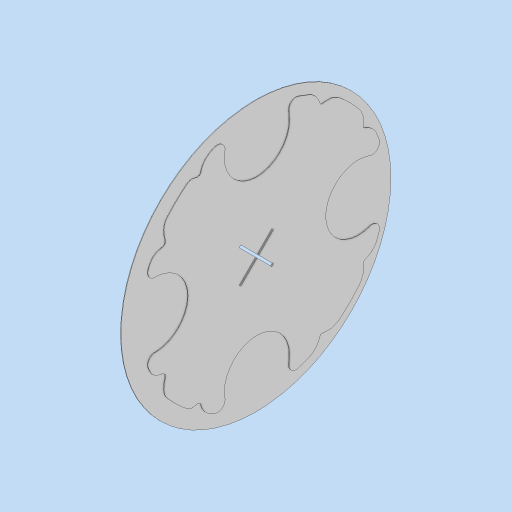
# Autodesk Inventor part: Sticker1
Saved by Autodesk Inventor 2024 (Build 280153000, 153)
## iProperties
Created: 2025-01-25
Part Number: Sticker1
Material: Generic
Document SubType Name: Modeling
Designer: Dmitry
Density: 1 g/cm^3
Appearance: Default
Author: Dmitry
Autodesk Inventor part; units mm, degrees
(part 1 of 2)
ref_plane "YZ Plane" through (0, 0, 0) normal (1, 0, 0) x (0, 1, 0)
ref_plane "XZ Plane" through (0, 0, 0) normal (0, 1, 0) x (-1, 0, 0)
ref_plane "XY Plane" through (0, 0, 0) normal (0, 0, 1) x (1, 0, 0)
sketch "Sketch1" plane through (0, 0, 0) normal (1, 0, 0) x (0, 1, 0)
  line L0 (61.7061, -10.6192) -> (60.2494, -12.386)
  line L1 (60.2494, -12.386) -> (59.1486, -14.4129)
  line L2 (59.1486, -14.4129) -> (58.4523, -16.6524)
  line L3 (58.4523, -16.6524) -> (58.211, -18.4561)
  line L4 (58.211, -18.4561) -> (58.211, -19.0583)
  line L5 (58.211, -19.0583) -> (58.211, -19.6593)
  line L6 (58.211, -19.6593) -> (58.4523, -21.4632)
  line L7 (58.4523, -21.4632) -> (59.1486, -23.7037)
  line L8 (59.1486, -23.7037) -> (60.2494, -25.7309)
  line L9 (60.2494, -25.7309) -> (61.7061, -27.4975)
  line L10 (61.7061, -39.6202) -> (60.2494, -41.3868)
  line L11 (60.2494, -41.3868) -> (59.1486, -43.4139)
  line L12 (59.1486, -43.4139) -> (58.4523, -45.6533)
  line L13 (58.4523, -45.6533) -> (58.211, -47.4571)
  line L14 (58.211, -47.4571) -> (58.211, -48.0593)
  line L15 (58.211, -48.0593) -> (58.211, -48.6601)
  line L16 (58.211, -48.6601) -> (58.4523, -50.464)
  line L17 (58.4523, -50.464) -> (59.1486, -52.7033)
  line L18 (59.1486, -52.7033) -> (60.2494, -54.7304)
  line L19 (60.2494, -54.7304) -> (61.7061, -56.497)
  line L20 (61.7061, 18.3803) -> (60.2494, 16.6135)
  line L21 (60.2494, 16.6135) -> (59.1486, 14.5863)
  line L22 (59.1486, 14.5863) -> (58.4523, 12.347)
  line L23 (58.4523, 12.347) -> (58.211, 10.5431)
  line L24 (58.211, 10.5431) -> (58.211, 9.9411)
  line L25 (58.211, 9.9411) -> (58.211, 9.3402)
  line L26 (58.211, 9.3402) -> (58.4523, 7.5363)
  line L27 (58.4523, 7.5363) -> (59.1486, 5.297)
  line L28 (59.1486, 5.297) -> (60.2494, 3.2701)
  line L29 (60.2494, 3.2701) -> (61.7061, 1.5032)
  line L30 (-65.1162, -39.6422) -> (-65.1135, -39.6381)
  line L31 (-65.1135, -39.6381) -> (-65.0777, -39.6023)
  line L32 (-65.0777, -39.6023) -> (-65.0735, -39.5995)
  line L33 (-65.0735, -39.5995) -> (-64.7194, -39.2412)
  line L34 (-64.7194, -39.2412) -> (-63.3482, -38.4723)
  line L35 (-63.3482, -38.4723) -> (-61.3997, -38.1637)
  line L36 (-61.3997, -38.1637) -> (-59.5007, -38.6666)
  line L37 (-59.5007, -38.6666) -> (-58.2302, -39.5816)
  line L38 (-58.2302, -39.5816) -> (-57.9229, -39.9771)
  line L39 (-57.9229, -39.9771) -> (-57.4888, -40.5366)
  line L40 (-57.4888, -40.5366) -> (-55.2495, -43.4098)
  line L41 (-55.2495, -43.4098) -> (-53.1783, -46.0363)
  line L42 (-53.1783, -46.0363) -> (-52.8283, -46.4746)
  line L43 (-52.8283, -46.4746) -> (-52.4672, -46.9265)
  line L44 (-52.4672, -46.9265) -> (-51.3813, -48.2853)
  line L45 (-51.3813, -48.2853) -> (-50.1039, -49.8893)
  line L46 (-50.1039, -49.8893) -> (-49.1268, -51.1364)
  line L47 (-49.1268, -51.1364) -> (-48.6749, -51.7276)
  line L48 (-48.6749, -51.7276) -> (-48.5784, -51.871)
  line L49 (-48.5784, -51.871) -> (-48.4159, -52.1093)
  line L50 (-48.4159, -52.1093) -> (-48.2889, -52.2968)
  line L51 (-48.2889, -52.2968) -> (-47.9058, -52.8618)
  line L52 (-47.9058, -52.8618) -> (-47.2886, -53.8057)
  line L53 (-47.2886, -53.8057) -> (-46.6341, -54.8682)
  line L54 (-46.6341, -54.8682) -> (-46.0138, -55.9775)
  line L55 (-46.0138, -55.9775) -> (-45.4999, -57.0593)
  line L56 (-45.4999, -57.0593) -> (-45.1621, -58.0432)
  line L57 (-45.1621, -58.0432) -> (-45.074, -58.8576)
  line L58 (-45.074, -58.8576) -> (-45.2051, -59.3261)
  line L59 (-45.2051, -59.3261) -> (-45.3028, -59.4281)
  line L60 (-45.3028, -59.4281) -> (-45.3153, -59.4405)
  line L61 (-45.3153, -59.4405) -> (-45.5137, -59.6321)
  line L62 (-45.5137, -59.6321) -> (-46.7098, -59.5907)
  line L63 (-46.7098, -59.5907) -> (-48.7809, -58.7446)
  line L64 (-48.7809, -58.7446) -> (-50.9527, -57.4727)
  line L65 (-50.9527, -57.4727) -> (-52.2302, -56.6321)
  line L66 (-52.2302, -56.6321) -> (-52.6505, -56.3468)
  line L67 (-52.6505, -56.3468) -> (-52.8903, -56.1828)
  line L68 (-52.8903, -56.1828) -> (-53.0322, -56.0864)
  line L69 (-53.0322, -56.0864) -> (-53.622, -55.6357)
  line L70 (-53.622, -55.6357) -> (-54.8636, -54.6615)
  line L71 (-54.8636, -54.6615) -> (-56.4635, -53.3895)
  line L72 (-56.4635, -53.3895) -> (-57.8168, -52.3064)
  line L73 (-57.8168, -52.3064) -> (-58.2674, -51.9467)
  line L74 (-58.2674, -51.9467) -> (-58.7056, -51.5967)
  line L75 (-58.7056, -51.5967) -> (-61.339, -49.52)
  line L76 (-61.339, -49.52) -> (-64.2219, -47.2738)
  line L77 (-64.2219, -47.2738) -> (-64.7841, -46.8383)
  line L78 (-64.7841, -46.8383) -> (-65.1796, -46.531)
  line L79 (-65.1796, -46.531) -> (-66.0946, -45.2591)
  line L80 (-66.0946, -45.2591) -> (-66.5976, -43.3616)
  line L81 (-66.5976, -43.3616) -> (-66.289, -41.413)
  line L82 (-66.289, -41.413) -> (-65.52, -40.0419)
  line L83 (-65.52, -40.0419) -> (-65.1617, -39.6877)
  line L84 (-65.1617, -39.6877) -> (-65.159, -39.6836)
  line L85 (-65.159, -39.6836) -> (-65.1204, -39.645)
  line L86 (-65.1204, -39.645) -> (-65.1162, -39.6422)
  line L87 (63.4051, 37.9784) -> (59.4061, 40.3805)
  line L88 (59.4061, 40.3805) -> (55.6728, 43.142)
  line L89 (55.6728, 43.142) -> (52.2278, 46.2372)
  line L90 (52.2278, 46.2372) -> (49.0983, 49.6436)
  line L91 (49.0983, 49.6436) -> (46.3063, 53.3355)
  line L92 (46.3063, 53.3355) -> (43.8771, 57.289)
  line L93 (43.8771, 57.289) -> (41.8334, 61.4823)
  line L94 (60.8986, 37.5649) -> (56.1567, 40.4534)
  line L95 (56.1567, 40.4534) -> (51.7274, 43.7716)
  line L96 (51.7274, 43.7716) -> (47.6391, 47.4897)
  line L97 (47.6391, 47.4897) -> (43.9213, 51.5783)
  line L98 (43.9213, 51.5783) -> (40.6025, 56.0073)
  line L99 (40.6025, 56.0073) -> (37.7145, 60.7493)
  line L100 (37.7145, 60.7493) -> (35.2848, 65.7724)
  line L101 (63.2179, 39.2809) -> (58.8176, 41.9609)
  line L102 (58.8176, 41.9609) -> (54.7056, 45.0409)
  line L103 (54.7056, 45.0409) -> (50.9118, 48.4915)
  line L104 (50.9118, 48.4915) -> (47.4613, 52.2852)
  line L105 (47.4613, 52.2852) -> (44.3813, 56.3972)
  line L106 (44.3813, 56.3972) -> (41.701, 60.7975)
  line L107 (41.701, 60.7975) -> (39.4465, 65.4594)
  line L108 (64.542, 40.6934) -> (60.4325, 43.1956)
  line L109 (60.4325, 43.1956) -> (56.5933, 46.0719)
  line L110 (56.5933, 46.0719) -> (53.0503, 49.2939)
  line L111 (53.0503, 49.2939) -> (49.8273, 52.8377)
  line L112 (49.8273, 52.8377) -> (46.9525, 56.6771)
  line L113 (46.9525, 56.6771) -> (44.4488, 60.7866)
  line L114 (44.4488, 60.7866) -> (42.3432, 65.1399)
  line L115 (64.542, 40.6947) -> (60.4325, 43.1971)
  line L116 (60.4325, 43.1971) -> (56.5933, 46.0731)
  line L117 (56.5933, 46.0731) -> (53.0503, 49.2949)
  line L118 (53.0503, 49.2949) -> (49.8288, 52.8377)
  line L119 (49.8288, 52.8377) -> (46.9525, 56.6771)
  line L120 (46.9525, 56.6771) -> (44.4503, 60.7866)
  line L121 (44.4503, 60.7866) -> (42.3447, 65.1409)
  line L122 (63.004, 46.765) -> (59.4269, 49.4109)
  line L123 (59.4269, 49.4109) -> (56.1249, 52.3764)
  line L124 (56.1249, 52.3764) -> (53.1247, 55.6408)
  line L125 (53.1247, 55.6408) -> (50.4486, 59.1795)
  line L126 (50.4486, 59.1795) -> (48.1214, 62.9692)
  line L127 (47.395, -6.0512) -> (47.395, -7.4304)
  line L128 (47.395, -7.4304) -> (47.1153, -11.5717)
  line L129 (47.1153, -11.5717) -> (46.2969, -16.9336)
  line L130 (46.2969, -16.9336) -> (44.9667, -22.1081)
  line L131 (44.9667, -22.1081) -> (43.1506, -27.0702)
  line L132 (43.1506, -27.0702) -> (40.8771, -31.7903)
  line L133 (40.8771, -31.7903) -> (38.172, -36.2427)
  line L134 (38.172, -36.2427) -> (35.063, -40.4001)
  line L135 (35.063, -40.4001) -> (31.5779, -44.2338)
  line L136 (31.5779, -44.2338) -> (27.7443, -47.7189)
  line L137 (27.7443, -47.7189) -> (23.5868, -50.8278)
  line L138 (23.5868, -50.8278) -> (19.1344, -53.5329)
  line L139 (19.1344, -53.5329) -> (14.4146, -55.8066)
  line L140 (14.4146, -55.8066) -> (9.4524, -57.6229)
  line L141 (9.4524, -57.6229) -> (4.2777, -58.9527)
  line L142 (4.2777, -58.9527) -> (-1.0845, -59.7713)
  line L143 (-1.0845, -59.7713) -> (-5.2255, -60.051)
  line L144 (-5.2255, -60.051) -> (-6.6047, -60.051)
  line L145 (-6.6047, -60.051) -> (-7.9854, -60.051)
  line L146 (-7.9854, -60.051) -> (-12.1264, -59.7713)
  line L147 (-12.1264, -59.7713) -> (-17.4886, -58.9527)
  line L148 (-17.4886, -58.9527) -> (-22.6631, -57.6229)
  line L149 (-22.6631, -57.6229) -> (-27.6252, -55.8066)
  line L150 (-27.6252, -55.8066) -> (-32.345, -53.5329)
  line L151 (-32.345, -53.5329) -> (-36.7977, -50.8278)
  line L152 (-36.7977, -50.8278) -> (-40.9551, -47.7189)
  line L153 (-40.9551, -47.7189) -> (-44.7887, -44.2338)
  line L154 (-44.7887, -44.2338) -> (-48.2739, -40.4001)
  line L155 (-48.2739, -40.4001) -> (-51.3827, -36.2427)
  line L156 (-51.3827, -36.2427) -> (-54.0878, -31.7903)
  line L157 (-54.0878, -31.7903) -> (-56.3616, -27.0702)
  line L158 (-56.3616, -27.0702) -> (-58.1778, -22.1081)
  line L159 (-58.1778, -22.1081) -> (-59.5076, -16.9336)
  line L160 (-59.5076, -16.9336) -> (-60.3262, -11.5717)
  line L161 (-60.3262, -11.5717) -> (-60.6045, -7.4304)
  line L162 (-60.6045, -7.4304) -> (-60.6045, -6.0512)
  line L163 (-60.6045, -6.0512) -> (-60.6045, -4.6702)
  line L164 (-60.6045, -4.6702) -> (-60.3262, -0.5295)
  line L165 (-60.3262, -0.5295) -> (-59.5076, 4.8324)
  line L166 (-59.5076, 4.8324) -> (-58.1778, 10.0069)
  line L167 (-58.1778, 10.0069) -> (-56.3616, 14.9696)
  line L168 (-56.3616, 14.9696) -> (-54.0878, 19.6894)
  line L169 (-54.0878, 19.6894) -> (-51.3827, 24.1418)
  line L170 (-51.3827, 24.1418) -> (-48.2739, 28.2992)
  line L171 (-48.2739, 28.2992) -> (-44.7887, 32.1344)
  line L172 (-44.7887, 32.1344) -> (-40.9551, 35.6193)
  line L173 (-40.9551, 35.6193) -> (-36.7977, 38.728)
  line L174 (-36.7977, 38.728) -> (-32.345, 41.4331)
  line L175 (-32.345, 41.4331) -> (-27.6252, 43.7071)
  line L176 (-27.6252, 43.7071) -> (-22.6631, 45.5232)
  line L177 (-22.6631, 45.5232) -> (-17.4886, 46.8532)
  line L178 (-17.4886, 46.8532) -> (-12.1264, 47.6716)
  line L179 (-12.1264, 47.6716) -> (-7.9854, 47.9499)
  line L180 (-7.9854, 47.9499) -> (-6.6047, 47.9499)
  line L181 (-6.6047, 47.9499) -> (-5.2255, 47.9499)
  line L182 (-5.2255, 47.9499) -> (-1.0845, 47.6716)
  line L183 (-1.0845, 47.6716) -> (4.2777, 46.8532)
  line L184 (4.2777, 46.8532) -> (9.4524, 45.5232)
  line L185 (9.4524, 45.5232) -> (14.4146, 43.7071)
  line L186 (14.4146, 43.7071) -> (19.1344, 41.4331)
  line L187 (19.1344, 41.4331) -> (23.5868, 38.728)
  line L188 (23.5868, 38.728) -> (27.7443, 35.6193)
  line L189 (27.7443, 35.6193) -> (31.5779, 32.1344)
  line L190 (31.5779, 32.1344) -> (35.063, 28.2992)
  line L191 (35.063, 28.2992) -> (38.172, 24.1418)
  line L192 (38.172, 24.1418) -> (40.8771, 19.6894)
  line L193 (40.8771, 19.6894) -> (43.1506, 14.9696)
  line L194 (43.1506, 14.9696) -> (44.9667, 10.0069)
  line L195 (44.9667, 10.0069) -> (46.2969, 4.8324)
  line L196 (46.2969, 4.8324) -> (47.1153, -0.5295)
  line L197 (47.1153, -0.5295) -> (47.395, -4.6702)
  line L198 (47.395, -4.6702) -> (47.395, -6.0512)
  line L199 (10.1675, -3.1226) -> (10.1675, -3.9677)
  line L200 (10.1675, -3.9677) -> (9.8256, -6.5021)
  line L201 (9.8256, -6.5021) -> (8.8487, -9.6504)
  line L202 (8.8487, -9.6504) -> (7.3026, -12.4993)
  line L203 (7.3026, -12.4993) -> (5.2546, -14.9808)
  line L204 (5.2546, -14.9808) -> (2.7728, -17.0286)
  line L205 (2.7728, -17.0286) -> (-0.0769, -18.5747)
  line L206 (-0.0769, -18.5747) -> (-3.2244, -19.5518)
  line L207 (-3.2244, -19.5518) -> (-5.7589, -19.8937)
  line L208 (-5.7589, -19.8937) -> (-6.6034, -19.8937)
  line L209 (-6.6034, -19.8937) -> (-7.4497, -19.8937)
  line L210 (-7.4497, -19.8937) -> (-9.9836, -19.5518)
  line L211 (-9.9836, -19.5518) -> (-13.1325, -18.5747)
  line L212 (-13.1325, -18.5747) -> (-15.9808, -17.0286)
  line L213 (-15.9808, -17.0286) -> (-18.4639, -14.9808)
  line L214 (-18.4639, -14.9808) -> (-20.5119, -12.4993)
  line L215 (-20.5119, -12.4993) -> (-22.058, -9.6504)
  line L216 (-22.058, -9.6504) -> (-23.0349, -6.5021)
  line L217 (-23.0349, -6.5021) -> (-23.3755, -3.9677)
  line L218 (-23.3755, -3.9677) -> (-23.3755, -3.1226)
  line L219 (-23.3755, -3.1226) -> (-23.3755, -2.2768)
  line L220 (-23.3755, -2.2768) -> (-23.0349, 0.2576)
  line L221 (-23.0349, 0.2576) -> (-22.058, 3.4047)
  line L222 (-22.058, 3.4047) -> (-20.5119, 6.2548)
  line L223 (-20.5119, 6.2548) -> (-18.4639, 8.7367)
  line L224 (-18.4639, 8.7367) -> (-15.9808, 10.7842)
  line L225 (-15.9808, 10.7842) -> (-13.1325, 12.3305)
  line L226 (-13.1325, 12.3305) -> (-9.9836, 13.3076)
  line L227 (-9.9836, 13.3076) -> (-7.4497, 13.648)
  line L228 (-7.4497, 13.648) -> (-6.6034, 13.648)
  line L229 (-6.6034, 13.648) -> (-5.7589, 13.648)
  line L230 (-5.7589, 13.648) -> (-3.2244, 13.3076)
  line L231 (-3.2244, 13.3076) -> (-0.0769, 12.3305)
  line L232 (-0.0769, 12.3305) -> (2.7728, 10.7842)
  line L233 (2.7728, 10.7842) -> (5.2546, 8.7367)
  line L234 (5.2546, 8.7367) -> (7.3026, 6.2548)
  line L235 (7.3026, 6.2548) -> (8.8487, 3.4047)
  line L236 (8.8487, 3.4047) -> (9.8256, 0.2576)
  line L237 (9.8256, 0.2576) -> (10.1675, -2.2768)
  line L238 (10.1675, -2.2768) -> (10.1675, -3.1226)
  line L239 (-15.0756, -11.7078) -> (-14.4512, -11.0852)
  line L240 (-13.2449, -9.8771) -> (0.639, 4.005)
  line L241 (1.2419, 4.6094) -> (1.8662, 5.2322)
  line L242 (1.8662, -11.7078) -> (1.2419, -11.0852)
  line L243 (0.0346, -9.878) -> (-13.8475, 4.0059)
  line L244 (-14.4512, 4.6094) -> (-15.0756, 5.2322)
  line L245 (43.4869, -21.0441) -> (43.4552, -21.1284)
  line L246 (43.4552, -21.1284) -> (43.3602, -21.3847)
  line L247 (43.3602, -21.3847) -> (43.1577, -21.9232)
  line L248 (43.1577, -21.9232) -> (42.9055, -22.5945)
  line L249 (42.9055, -22.5945) -> (42.6271, -23.3319)
  line L250 (42.6271, -23.3319) -> (42.3475, -24.0677)
  line L251 (42.3475, -24.0677) -> (42.0925, -24.736)
  line L252 (42.0925, -24.736) -> (41.8857, -25.2737)
  line L253 (41.8857, -25.2737) -> (41.7866, -25.5269)
  line L254 (41.7866, -25.5269) -> (41.7534, -25.6113)
  line L255 (41.7534, -25.6113) -> (41.5921, -26.0039)
  line L256 (41.5921, -26.0039) -> (40.9088, -27.1035)
  line L257 (40.9088, -27.1035) -> (39.7386, -28.3367)
  line L258 (39.7386, -28.3367) -> (38.3096, -29.2945)
  line L259 (38.3096, -29.2945) -> (37.1014, -29.8348)
  line L260 (37.1014, -29.8348) -> (36.6823, -29.9602)
  line L261 (36.6823, -29.9602) -> (36.5898, -29.9864)
  line L262 (36.5898, -29.9864) -> (35.8994, -30.4756)
  line L263 (35.8994, -30.4756) -> (35.8568, -30.5472)
  line L264 (35.8568, -30.5472) -> (35.8098, -30.6217)
  line L265 (35.8098, -30.6217) -> (35.7135, -31.516)
  line L266 (35.7135, -31.516) -> (35.7381, -31.6166)
  line L267 (35.7381, -31.6166) -> (35.8804, -32.1967)
  line L268 (35.8804, -32.1967) -> (35.8169, -35.1098)
  line L269 (35.8169, -35.1098) -> (34.7186, -37.8081)
  line L270 (34.7186, -37.8081) -> (34.345, -38.2808)
  line L271 (34.345, -38.2808) -> (33.6932, -39.1035)
  line L272 (33.6932, -39.1035) -> (30.1545, -42.9661)
  line L273 (30.1545, -42.9661) -> (26.2629, -46.4746)
  line L274 (26.2629, -46.4746) -> (25.4359, -47.1195)
  line L275 (25.4359, -47.1195) -> (24.9856, -47.4695)
  line L276 (24.9856, -47.4695) -> (22.4097, -48.4989)
  line L277 (22.4097, -48.4989) -> (19.6015, -48.627)
  line L278 (19.6015, -48.627) -> (19.0351, -48.5278)
  line L279 (19.0351, -48.5278) -> (18.9551, -48.514)
  line L280 (18.9551, -48.514) -> (18.233, -48.6133)
  line L281 (18.233, -48.6133) -> (18.171, -48.6491)
  line L282 (18.171, -48.6491) -> (18.1022, -48.6863)
  line L283 (18.1022, -48.6863) -> (17.6307, -49.3064)
  line L284 (17.6307, -49.3064) -> (17.6046, -49.3905)
  line L285 (17.6046, -49.3905) -> (17.4781, -49.7818)
  line L286 (17.4781, -49.7818) -> (16.9432, -50.9105)
  line L287 (16.9432, -50.9105) -> (16.0021, -52.2513)
  line L288 (16.0021, -52.2513) -> (14.7948, -53.3579)
  line L289 (14.7948, -53.3579) -> (13.7227, -54.0166)
  line L290 (13.7227, -54.0166) -> (13.3409, -54.175)
  line L291 (13.3409, -54.175) -> (13.0943, -54.277)
  line L292 (13.0943, -54.277) -> (10.596, -55.2223)
  line L293 (10.596, -55.2223) -> (10.3425, -55.3106)
  line L294 (10.3425, -55.3106) -> (10.1233, -55.385)
  line L295 (10.1233, -55.385) -> (9.4235, -55.4814)
  line L296 (9.4235, -55.4814) -> (8.5576, -55.3836)
  line L297 (8.5576, -55.3836) -> (7.7791, -55.0515)
  line L298 (7.7791, -55.0515) -> (7.1261, -54.5264)
  line L299 (7.1261, -54.5264) -> (6.6313, -53.8443)
  line L300 (6.6313, -53.8443) -> (6.3323, -53.0464)
  line L301 (6.3323, -53.0464) -> (6.2622, -52.1686)
  line L302 (6.2622, -52.1686) -> (6.3793, -51.4686)
  line L303 (6.3793, -51.4686) -> (6.4603, -51.2522)
  line L304 (6.4603, -51.2522) -> (6.5982, -50.8774)
  line L305 (6.5982, -50.8774) -> (7.093, -48.9247)
  line L306 (7.093, -48.9247) -> (7.3135, -47.0726)
  line L307 (7.3135, -47.0726) -> (7.3135, -46.4566)
  line L308 (7.3135, -46.4566) -> (7.3135, -45.7621)
  line L309 (7.3135, -45.7621) -> (7.0336, -43.6785)
  line L310 (7.0336, -43.6785) -> (6.2343, -41.0892)
  line L311 (6.2343, -41.0892) -> (4.9696, -38.741)
  line L312 (4.9696, -38.741) -> (3.294, -36.6905)
  line L313 (3.294, -36.6905) -> (1.2625, -34.9927)
  line L314 (1.2625, -34.9927) -> (-1.0693, -33.7017)
  line L315 (-1.0693, -33.7017) -> (-3.6458, -32.8718)
  line L316 (-3.6458, -32.8718) -> (-5.7213, -32.5701)
  line L317 (-5.7213, -32.5701) -> (-6.4132, -32.562)
  line L318 (-6.4132, -32.562) -> (-6.4614, -32.562)
  line L319 (-6.4614, -32.562) -> (-6.5691, -32.5648)
  line L320 (-6.5691, -32.5648) -> (-6.6047, -32.5648)
  line L321 (-6.6047, -32.5648) -> (-6.6529, -32.5648)
  line L322 (-6.6529, -32.5648) -> (-6.7604, -32.562)
  line L323 (-6.7604, -32.562) -> (-6.7962, -32.562)
  line L324 (-6.7962, -32.562) -> (-7.4894, -32.5701)
  line L325 (-7.4894, -32.5701) -> (-9.5635, -32.8718)
  line L326 (-9.5635, -32.8718) -> (-12.1401, -33.7017)
  line L327 (-12.1401, -33.7017) -> (-14.4721, -34.9927)
  line L328 (-14.4721, -34.9927) -> (-16.5033, -36.6905)
  line L329 (-16.5033, -36.6905) -> (-18.1789, -38.741)
  line L330 (-18.1789, -38.741) -> (-19.4441, -41.0892)
  line L331 (-19.4441, -41.0892) -> (-20.2432, -43.6785)
  line L332 (-20.2432, -43.6785) -> (-20.5213, -45.7621)
  line L333 (-20.5213, -45.7621) -> (-20.5213, -46.4566)
  line L334 (-20.5213, -46.4566) -> (-20.5213, -47.0726)
  line L335 (-20.5213, -47.0726) -> (-20.3024, -48.9247)
  line L336 (-20.3024, -48.9247) -> (-19.8063, -50.8774)
  line L337 (-19.8063, -50.8774) -> (-19.6684, -51.2522)
  line L338 (-19.6684, -51.2522) -> (-19.5886, -51.4686)
  line L339 (-19.5886, -51.4686) -> (-19.4716, -52.1686)
  line L340 (-19.4716, -52.1686) -> (-19.5417, -53.0464)
  line L341 (-19.5417, -53.0464) -> (-19.8409, -53.8443)
  line L342 (-19.8409, -53.8443) -> (-20.3354, -54.5264)
  line L343 (-20.3354, -54.5264) -> (-20.9889, -55.0515)
  line L344 (-20.9889, -55.0515) -> (-21.7675, -55.3836)
  line L345 (-21.7675, -55.3836) -> (-22.6328, -55.4814)
  line L346 (-22.6328, -55.4814) -> (-23.3326, -55.385)
  line L347 (-23.3326, -55.385) -> (-23.5503, -55.3106)
  line L348 (-23.5503, -55.3106) -> (-23.804, -55.2223)
  line L349 (-23.804, -55.2223) -> (-26.3039, -54.277)
  line L350 (-26.3039, -54.277) -> (-26.549, -54.175)
  line L351 (-26.549, -54.175) -> (-26.932, -54.0166)
  line L352 (-26.932, -54.0166) -> (-28.0042, -53.3579)
  line L353 (-28.0042, -53.3579) -> (-29.2099, -52.2513)
  line L354 (-29.2099, -52.2513) -> (-30.1525, -50.9105)
  line L355 (-30.1525, -50.9105) -> (-30.6859, -49.7818)
  line L356 (-30.6859, -49.7818) -> (-30.8127, -49.3905)
  line L357 (-30.8127, -49.3905) -> (-30.8401, -49.3064)
  line L358 (-30.8401, -49.3064) -> (-31.31, -48.6863)
  line L359 (-31.31, -48.6863) -> (-31.3778, -48.6491)
  line L360 (-31.3778, -48.6491) -> (-31.441, -48.6133)
  line L361 (-31.441, -48.6133) -> (-32.1632, -48.514)
  line L362 (-32.1632, -48.514) -> (-32.2432, -48.5292)
  line L363 (-32.2432, -48.5292) -> (-32.8093, -48.6285)
  line L364 (-32.8093, -48.6285) -> (-35.6193, -48.5003)
  line L365 (-35.6193, -48.5003) -> (-38.1949, -47.4695)
  line L366 (-38.1949, -47.4695) -> (-38.644, -47.1195)
  line L367 (-38.644, -47.1195) -> (-39.4723, -46.4746)
  line L368 (-39.4723, -46.4746) -> (-43.3638, -42.9661)
  line L369 (-43.3638, -42.9661) -> (-46.9013, -39.1035)
  line L370 (-46.9013, -39.1035) -> (-47.5518, -38.282)
  line L371 (-47.5518, -38.282) -> (-47.9267, -37.8093)
  line L372 (-47.9267, -37.8093) -> (-49.025, -35.1098)
  line L373 (-49.025, -35.1098) -> (-49.0897, -32.1967)
  line L374 (-49.0897, -32.1967) -> (-48.9462, -31.6166)
  line L375 (-48.9462, -31.6166) -> (-48.9216, -31.516)
  line L376 (-48.9216, -31.516) -> (-49.0194, -30.6217)
  line L377 (-49.0194, -30.6217) -> (-49.0648, -30.5472)
  line L378 (-49.0648, -30.5472) -> (-49.109, -30.4756)
  line L379 (-49.109, -30.4756) -> (-49.7993, -29.9864)
  line L380 (-49.7993, -29.9864) -> (-49.8903, -29.9602)
  line L381 (-49.8903, -29.9602) -> (-50.3092, -29.8348)
  line L382 (-50.3092, -29.8348) -> (-51.5178, -29.296)
  line L383 (-51.5178, -29.296) -> (-52.9482, -28.3382)
  line L384 (-52.9482, -28.3382) -> (-54.1167, -27.1035)
  line L385 (-54.1167, -27.1035) -> (-54.8003, -26.0039)
  line L386 (-54.8003, -26.0039) -> (-54.9601, -25.6113)
  line L387 (-54.9601, -25.6113) -> (-54.9946, -25.5269)
  line L388 (-54.9946, -25.5269) -> (-55.0938, -25.2737)
  line L389 (-55.0938, -25.2737) -> (-55.3005, -24.736)
  line L390 (-55.3005, -24.736) -> (-55.5568, -24.0677)
  line L391 (-55.5568, -24.0677) -> (-55.8365, -23.3319)
  line L392 (-55.8365, -23.3319) -> (-56.1149, -22.5945)
  line L393 (-56.1149, -22.5945) -> (-56.3671, -21.9232)
  line L394 (-56.3671, -21.9232) -> (-56.5696, -21.3847)
  line L395 (-56.5696, -21.3847) -> (-56.6647, -21.1284)
  line L396 (-56.6647, -21.1284) -> (-56.695, -21.0441)
  line L397 (-56.695, -21.0441) -> (-56.7694, -20.8432)
  line L398 (-56.7694, -20.8432) -> (-56.8811, -20.2011)
  line L399 (-56.8811, -20.2011) -> (-56.837, -19.3877)
  line L400 (-56.837, -19.3877) -> (-56.5889, -18.6354)
  line L401 (-56.5889, -18.6354) -> (-56.1631, -17.9768)
  line L402 (-56.1631, -17.9768) -> (-55.5885, -17.4419)
  line L403 (-55.5885, -17.4419) -> (-54.8912, -17.0659)
  line L404 (-54.8912, -17.0659) -> (-54.0974, -16.8785)
  line L405 (-54.0974, -16.8785) -> (-53.4443, -16.8772)
  line L406 (-53.4443, -16.8772) -> (-53.2334, -16.9143)
  line L407 (-53.2334, -16.9143) -> (-53.046, -16.9473)
  line L408 (-53.046, -16.9473) -> (-52.4727, -17.0052)
  line L409 (-52.4727, -17.0052) -> (-51.5053, -17.0715)
  line L410 (-51.5053, -17.0715) -> (-50.5311, -17.1114)
  line L411 (-50.5311, -17.1114) -> (-49.9441, -17.1251)
  line L412 (-49.9441, -17.1251) -> (-49.747, -17.1251)
  line L413 (-49.747, -17.1251) -> (-49.0471, -17.1238)
  line L414 (-49.0471, -17.1238) -> (-46.9439, -16.8317)
  line L415 (-46.9439, -16.8317) -> (-44.3285, -16.0004)
  line L416 (-44.3285, -16.0004) -> (-41.9582, -14.6903)
  line L417 (-41.9582, -14.6903) -> (-39.8939, -12.9605)
  line L418 (-39.8939, -12.9605) -> (-38.1949, -10.8714)
  line L419 (-38.1949, -10.8714) -> (-36.9175, -8.4835)
  line L420 (-36.9175, -8.4835) -> (-36.1223, -5.8567)
  line L421 (-36.1223, -5.8567) -> (-35.8606, -3.75)
  line L422 (-35.8606, -3.75) -> (-35.8688, -3.0497)
  line L423 (-35.8688, -3.0497) -> (-35.8784, -2.3568)
  line L424 (-35.8784, -2.3568) -> (-36.183, -0.2829)
  line L425 (-36.183, -0.2829) -> (-37.0123, 2.2929)
  line L426 (-37.0123, 2.2929) -> (-38.3039, 4.6219)
  line L427 (-38.3039, 4.6219) -> (-40.0016, 6.6518)
  line L428 (-40.0016, 6.6518) -> (-42.0519, 8.3259)
  line L429 (-42.0519, 8.3259) -> (-44.3989, 9.5911)
  line L430 (-44.3989, 9.5911) -> (-46.9881, 10.3887)
  line L431 (-46.9881, 10.3887) -> (-49.0704, 10.6671)
  line L432 (-49.0704, 10.6671) -> (-49.7635, 10.6671)
  line L433 (-49.7635, 10.6671) -> (-50.4002, 10.6671)
  line L434 (-50.4002, 10.6671) -> (-52.102, 10.4715)
  line L435 (-52.102, 10.4715) -> (-52.3074, 10.4329)
  line L436 (-52.3074, 10.4329) -> (-52.5141, 10.3958)
  line L437 (-52.5141, 10.3958) -> (-53.1562, 10.393)
  line L438 (-53.1562, 10.393) -> (-53.9403, 10.5749)
  line L439 (-53.9403, 10.5749) -> (-54.6335, 10.9454)
  line L440 (-54.6335, 10.9454) -> (-55.2068, 11.4735)
  line L441 (-55.2068, 11.4735) -> (-55.634, 12.125)
  line L442 (-55.634, 12.125) -> (-55.8875, 12.8695)
  line L443 (-55.8875, 12.8695) -> (-55.9413, 13.6726)
  line L444 (-55.9413, 13.6726) -> (-55.8365, 14.3066)
  line L445 (-55.8365, 14.3066) -> (-55.7649, 14.5035)
  line L446 (-55.7649, 14.5035) -> (-55.7332, 14.5944)
  line L447 (-55.7332, 14.5944) -> (-55.3997, 15.4915)
  line L448 (-55.3997, 15.4915) -> (-55.3652, 15.5812)
  line L449 (-55.3652, 15.5812) -> (-55.193, 16.0318)
  line L450 (-55.193, 16.0318) -> (-54.4654, 17.3026)
  line L451 (-54.4654, 17.3026) -> (-53.2017, 18.759)
  line L452 (-53.2017, 18.759) -> (-51.6266, 19.8672)
  line L453 (-51.6266, 19.8672) -> (-50.2651, 20.4377)
  line L454 (-50.2651, 20.4377) -> (-49.7911, 20.5423)
  line L455 (-49.7911, 20.5423) -> (-49.6505, 20.5738)
  line L456 (-49.6505, 20.5738) -> (-49.0539, 20.8359)
  line L457 (-49.0539, 20.8359) -> (-48.6211, 21.2423)
  line L458 (-48.6211, 21.2423) -> (-48.5632, 21.3442)
  line L459 (-48.5632, 21.3442) -> (-48.5109, 21.4395)
  line L460 (-48.5109, 21.4395) -> (-48.391, 21.9685)
  line L461 (-48.391, 21.9685) -> (-48.453, 22.5499)
  line L462 (-48.453, 22.5499) -> (-48.4916, 22.6714)
  line L463 (-48.4916, 22.6714) -> (-48.6114, 23.0475)
  line L464 (-48.6114, 23.0475) -> (-48.836, 24.2187)
  line L465 (-48.836, 24.2187) -> (-48.7052, 25.3653)
  line L466 (-48.7052, 25.3653) -> (-48.1182, 26.4293)
  line L467 (-48.1182, 26.4293) -> (-47.3547, 27.4049)
  line L468 (-47.3547, 27.4049) -> (-47.0943, 27.7247)
  line L469 (-47.0943, 27.7247) -> (-46.5403, 28.4054)
  line L470 (-46.5403, 28.4054) -> (-43.5693, 31.634)
  line L471 (-43.5693, 31.634) -> (-40.3501, 34.6147)
  line L472 (-40.3501, 34.6147) -> (-39.6706, 35.1715)
  line L473 (-39.6706, 35.1715) -> (-39.3097, 35.4691)
  line L474 (-39.3097, 35.4691) -> (-38.0075, 36.096)
  line L475 (-38.0075, 36.096) -> (-36.1609, 36.427)
  line L476 (-36.1609, 36.427) -> (-34.218, 36.3012)
  line L477 (-34.218, 36.3012) -> (-32.7433, 35.9939)
  line L478 (-32.7433, 35.9939) -> (-32.2625, 35.8537)
  line L479 (-32.2625, 35.8537) -> (-32.1136, 35.811)
  line L480 (-32.1136, 35.811) -> (-31.408, 35.7488)
  line L481 (-31.408, 35.7488) -> (-30.7837, 35.9086)
  line L482 (-30.7837, 35.9086) -> (-30.6737, 35.9749)
  line L483 (-30.6737, 35.9749) -> (-30.566, 36.0409)
  line L484 (-30.566, 36.0409) -> (-30.1431, 36.5095)
  line L485 (-30.1431, 36.5095) -> (-29.8937, 37.1405)
  line L486 (-29.8937, 37.1405) -> (-29.8729, 37.288)
  line L487 (-29.8729, 37.288) -> (-29.7875, 37.9083)
  line L488 (-29.7875, 37.9083) -> (-29.2198, 39.7231)
  line L489 (-29.2198, 39.7231) -> (-28.1299, 41.2748)
  line L490 (-28.1299, 41.2748) -> (-26.6689, 42.2601)
  line L491 (-26.6689, 42.2601) -> (-25.3461, 42.8265)
  line L492 (-25.3461, 42.8265) -> (-24.897, 42.9947)
  line L493 (-24.897, 42.9947) -> (-24.8818, 43.0015)
  line L494 (-24.8818, 43.0015) -> (-24.7177, 43.0622)
  line L495 (-24.7177, 43.0622) -> (-24.7012, 43.0676)
  line L496 (-24.7012, 43.0676) -> (-24.5206, 43.1354)
  line L497 (-24.5206, 43.1354) -> (-23.9404, 43.2469)
  line L498 (-23.9404, 43.2469) -> (-23.1896, 43.2329)
  line L499 (-23.1896, 43.2329) -> (-22.4797, 43.047)
  line L500 (-22.4797, 43.047) -> (-21.8363, 42.7038)
  line L501 (-21.8363, 42.7038) -> (-21.2892, 42.2255)
  line L502 (-21.2892, 42.2255) -> (-20.866, 41.6289)
  line L503 (-20.866, 41.6289) -> (-20.593, 40.9342)
  line L504 (-20.593, 40.9342) -> (-20.4995, 40.3531)
  line L505 (-20.4995, 40.3531) -> (-20.4995, 40.1585)
  line L506 (-20.4995, 40.1585) -> (-20.501, 40.0719)
  line L507 (-20.501, 40.0719) -> (-20.4746, 39.1956)
  line L508 (-20.4746, 39.1956) -> (-20.4677, 39.1072)
  line L509 (-20.4677, 39.1072) -> (-20.4251, 38.4747)
  line L510 (-20.4251, 38.4747) -> (-20.0585, 36.5908)
  line L511 (-20.0585, 36.5908) -> (-19.2137, 34.2413)
  line L512 (-19.2137, 34.2413) -> (-17.9775, 32.1054)
  line L513 (-17.9775, 32.1054) -> (-16.3943, 30.2271)
  line L514 (-16.3943, 30.2271) -> (-14.5104, 28.6533)
  line L515 (-14.5104, 28.6533) -> (-12.3692, 27.4267)
  line L516 (-12.3692, 27.4267) -> (-10.0167, 26.5931)
  line L517 (-10.0167, 26.5931) -> (-8.1302, 26.2362)
  line L518 (-8.1302, 26.2362) -> (-7.4962, 26.1964)
  line L519 (-7.4962, 26.1964) -> (-7.4218, 26.192)
  line L520 (-7.4218, 26.192) -> (-6.8099, 26.1702)
  line L521 (-6.8099, 26.1702) -> (-6.6047, 26.1702)
  line L522 (-6.6047, 26.1702) -> (-6.3814, 26.1702)
  line L523 (-6.3814, 26.1702) -> (-5.7863, 26.192)
  line L524 (-5.7863, 26.192) -> (-5.7103, 26.1964)
  line L525 (-5.7103, 26.1964) -> (-5.0779, 26.2362)
  line L526 (-5.0779, 26.2362) -> (-3.1912, 26.5931)
  line L527 (-3.1912, 26.5931) -> (-0.8389, 27.4267)
  line L528 (-0.8389, 27.4267) -> (1.3011, 28.6533)
  line L529 (1.3011, 28.6533) -> (3.185, 30.2271)
  line L530 (3.185, 30.2271) -> (4.7667, 32.1054)
  line L531 (4.7667, 32.1054) -> (6.0029, 34.2413)
  line L532 (6.0029, 34.2413) -> (6.8492, 36.5908)
  line L533 (6.8492, 36.5908) -> (7.2142, 38.4747)
  line L534 (7.2142, 38.4747) -> (7.2584, 39.1072)
  line L535 (7.2584, 39.1072) -> (7.2637, 39.1956)
  line L536 (7.2637, 39.1956) -> (7.2917, 40.0719)
  line L537 (7.2917, 40.0719) -> (7.2917, 40.1585)
  line L538 (7.2917, 40.1585) -> (7.2901, 40.3531)
  line L539 (7.2901, 40.3531) -> (7.3836, 40.9342)
  line L540 (7.3836, 40.9342) -> (7.6567, 41.6289)
  line L541 (7.6567, 41.6289) -> (8.0796, 42.2255)
  line L542 (8.0796, 42.2255) -> (8.6282, 42.7038)
  line L543 (8.6282, 42.7038) -> (9.2703, 43.047)
  line L544 (9.2703, 43.047) -> (9.9815, 43.2329)
  line L545 (9.9815, 43.2329) -> (10.7311, 43.2469)
  line L546 (10.7311, 43.2469) -> (11.3112, 43.1354)
  line L547 (11.3112, 43.1354) -> (11.4946, 43.0676)
  line L548 (11.4946, 43.0676) -> (11.5098, 43.0622)
  line L549 (11.5098, 43.0622) -> (11.6724, 43.0015)
  line L550 (11.6724, 43.0015) -> (11.6887, 42.9947)
  line L551 (11.6887, 42.9947) -> (12.1433, 42.8252)
  line L552 (12.1433, 42.8252) -> (13.4748, 42.2187)
  line L553 (13.4748, 42.2187) -> (14.9602, 41.1618)
  line L554 (14.9602, 41.1618) -> (16.0542, 39.5949)
  line L555 (16.0542, 39.5949) -> (16.5919, 37.875)
  line L556 (16.5919, 37.875) -> (16.6648, 37.288)
  line L557 (16.6648, 37.288) -> (16.6828, 37.1405)
  line L558 (16.6828, 37.1405) -> (16.931, 36.5095)
  line L559 (16.931, 36.5095) -> (17.3567, 36.0409)
  line L560 (17.3567, 36.0409) -> (17.4654, 35.9749)
  line L561 (17.4654, 35.9749) -> (17.5743, 35.9086)
  line L562 (17.5743, 35.9086) -> (18.1997, 35.7488)
  line L563 (18.1997, 35.7488) -> (18.9043, 35.811)
  line L564 (18.9043, 35.811) -> (19.0542, 35.8537)
  line L565 (19.0542, 35.8537) -> (19.534, 35.9939)
  line L566 (19.534, 35.9939) -> (21.0082, 36.3012)
  line L567 (21.0082, 36.3012) -> (22.9528, 36.427)
  line L568 (22.9528, 36.427) -> (24.7981, 36.096)
  line L569 (24.7981, 36.096) -> (26.1004, 35.4691)
  line L570 (26.1004, 35.4691) -> (26.4626, 35.1715)
  line L571 (26.4626, 35.1715) -> (27.1405, 34.6147)
  line L572 (27.1405, 34.6147) -> (30.3597, 31.634)
  line L573 (30.3597, 31.634) -> (33.3307, 28.4054)
  line L574 (33.3307, 28.4054) -> (33.886, 27.7247)
  line L575 (33.886, 27.7247) -> (34.1468, 27.4049)
  line L576 (34.1468, 27.4049) -> (34.9088, 26.4293)
  line L577 (34.9088, 26.4293) -> (35.4958, 25.3653)
  line L578 (35.4958, 25.3653) -> (35.6266, 24.2187)
  line L579 (35.6266, 24.2187) -> (35.4018, 23.0475)
  line L580 (35.4018, 23.0475) -> (35.2835, 22.6714)
  line L581 (35.2835, 22.6714) -> (35.2449, 22.5499)
  line L582 (35.2449, 22.5499) -> (35.1814, 21.9685)
  line L583 (35.1814, 21.9685) -> (35.3028, 21.4395)
  line L584 (35.3028, 21.4395) -> (35.3564, 21.3442)
  line L585 (35.3564, 21.3442) -> (35.413, 21.2423)
  line L586 (35.413, 21.2423) -> (35.8443, 20.8359)
  line L587 (35.8443, 20.8359) -> (36.441, 20.5738)
  line L588 (36.441, 20.5738) -> (36.5817, 20.5423)
  line L589 (36.5817, 20.5423) -> (37.0544, 20.4377)
  line L590 (37.0544, 20.4377) -> (38.4158, 19.8672)
  line L591 (38.4158, 19.8672) -> (39.9924, 18.759)
  line L592 (39.9924, 18.759) -> (41.256, 17.3038)
  line L593 (41.256, 17.3038) -> (41.9835, 16.0318)
  line L594 (41.9835, 16.0318) -> (42.1572, 15.5812)
  line L595 (42.1572, 15.5812) -> (42.1915, 15.4915)
  line L596 (42.1915, 15.4915) -> (42.5238, 14.5944)
  line L597 (42.5238, 14.5944) -> (42.5568, 14.5035)
  line L598 (42.5568, 14.5035) -> (42.6271, 14.3066)
  line L599 (42.6271, 14.3066) -> (42.7315, 13.6726)
  line L600 (42.7315, 13.6726) -> (42.6795, 12.8695)
  line L601 (42.6795, 12.8695) -> (42.4257, 12.125)
  line L602 (42.4257, 12.125) -> (41.9972, 11.4735)
  line L603 (41.9972, 11.4735) -> (41.4239, 10.9454)
  line L604 (41.4239, 10.9454) -> (40.731, 10.5749)
  line L605 (40.731, 10.5749) -> (39.9469, 10.393)
  line L606 (39.9469, 10.393) -> (39.3048, 10.3958)
  line L607 (39.3048, 10.3958) -> (39.0993, 10.4329)
  line L608 (39.0993, 10.4329) -> (38.8926, 10.4715)
  line L609 (38.8926, 10.4715) -> (37.1397, 10.6671)
  line L610 (37.1397, 10.6671) -> (36.5555, 10.6671)
  line L611 (36.5555, 10.6671) -> (35.8608, 10.6671)
  line L612 (35.8608, 10.6671) -> (33.7788, 10.3887)
  line L613 (33.7788, 10.3887) -> (31.1895, 9.5911)
  line L614 (31.1895, 9.5911) -> (28.8423, 8.3259)
  line L615 (28.8423, 8.3259) -> (26.792, 6.6518)
  line L616 (26.792, 6.6518) -> (25.0943, 4.6219)
  line L617 (25.0943, 4.6219) -> (23.8029, 2.2929)
  line L618 (23.8029, 2.2929) -> (22.9736, -0.2829)
  line L619 (22.9736, -0.2829) -> (22.6688, -2.3568)
  line L620 (22.6688, -2.3568) -> (22.6607, -3.0497)
  line L621 (22.6607, -3.0497) -> (22.651, -3.75)
  line L622 (22.651, -3.75) -> (22.9129, -5.8567)
  line L623 (22.9129, -5.8567) -> (23.7082, -8.4835)
  line L624 (23.7082, -8.4835) -> (24.9856, -10.8714)
  line L625 (24.9856, -10.8714) -> (26.6846, -12.9605)
  line L626 (26.6846, -12.9605) -> (28.7488, -14.6903)
  line L627 (28.7488, -14.6903) -> (31.1192, -15.9991)
  line L628 (31.1192, -15.9991) -> (33.7348, -16.8302)
  line L629 (33.7348, -16.8302) -> (35.8377, -17.1223)
  line L630 (35.8377, -17.1223) -> (36.539, -17.1238)
  line L631 (36.539, -17.1238) -> (36.7333, -17.1238)
  line L632 (36.7333, -17.1238) -> (37.3218, -17.1099)
  line L633 (37.3218, -17.1099) -> (38.2959, -17.0715)
  line L634 (38.2959, -17.0715) -> (39.2632, -17.0052)
  line L635 (39.2632, -17.0052) -> (39.8364, -16.9473)
  line L636 (39.8364, -16.9473) -> (40.0254, -16.9143)
  line L637 (40.0254, -16.9143) -> (40.2347, -16.8772)
  line L638 (40.2347, -16.8772) -> (40.888, -16.8785)
  line L639 (40.888, -16.8785) -> (41.6817, -17.0659)
  line L640 (41.6817, -17.0659) -> (42.379, -17.4419)
  line L641 (42.379, -17.4419) -> (42.9535, -17.9768)
  line L642 (42.9535, -17.9768) -> (43.3792, -18.6354)
  line L643 (43.3792, -18.6354) -> (43.6276, -19.3877)
  line L644 (43.6276, -19.3877) -> (43.6718, -20.2011)
  line L645 (43.6718, -20.2011) -> (43.5601, -20.8432)
  line L646 (43.5601, -20.8432) -> (43.4869, -21.0441)
  line L647 (-6.6034, 54.4404) -> (-6.6047, 54.4404)
  line L648 (-6.6047, 54.4404) -> (-8.0751, 54.4404)
  line L649 (-8.0751, 54.4404) -> (-12.4848, 54.1445)
  line L650 (-12.4848, 54.1445) -> (-18.1942, 53.2735)
  line L651 (-18.1942, 53.2735) -> (-23.7034, 51.8567)
  line L652 (-23.7034, 51.8567) -> (-28.9866, 49.9235)
  line L653 (-28.9866, 49.9235) -> (-34.0123, 47.5009)
  line L654 (-34.0123, 47.5009) -> (-38.7545, 44.6205)
  line L655 (-38.7545, 44.6205) -> (-43.1807, 41.3106)
  line L656 (-43.1807, 41.3106) -> (-47.2637, 37.5994)
  line L657 (-47.2637, 37.5994) -> (-50.9748, 33.5164)
  line L658 (-50.9748, 33.5164) -> (-54.2848, 29.0902)
  line L659 (-54.2848, 29.0902) -> (-57.1649, 24.3498)
  line L660 (-57.1649, 24.3498) -> (-59.5862, 19.3229)
  line L661 (-59.5862, 19.3229) -> (-61.5209, 14.0407)
  line L662 (-61.5209, 14.0407) -> (-62.9376, 8.5299)
  line L663 (-62.9376, 8.5299) -> (-63.8085, 2.8205)
  line L664 (-63.8085, 2.8205) -> (-64.1048, -1.5892)
  line L665 (-64.1048, -1.5892) -> (-64.1048, -3.0596)
  line L666 (-64.1048, -3.0596) -> (-64.1048, -4.5285)
  line L667 (-64.1048, -4.5285) -> (-63.8085, -8.9382)
  line L668 (-63.8085, -8.9382) -> (-62.9376, -14.6473)
  line L669 (-62.9376, -14.6473) -> (-61.5209, -20.1584)
  line L670 (-61.5209, -20.1584) -> (-59.5862, -25.4401)
  line L671 (-59.5862, -25.4401) -> (-57.1649, -30.4672)
  line L672 (-57.1649, -30.4672) -> (-54.2848, -35.2076)
  line L673 (-54.2848, -35.2076) -> (-50.9748, -39.634)
  line L674 (-50.9748, -39.634) -> (-47.2637, -43.7171)
  line L675 (-47.2637, -43.7171) -> (-43.1807, -47.4282)
  line L676 (-43.1807, -47.4282) -> (-38.7545, -50.7382)
  line L677 (-38.7545, -50.7382) -> (-34.0123, -53.6183)
  line L678 (-34.0123, -53.6183) -> (-28.9866, -56.0409)
  line L679 (-28.9866, -56.0409) -> (-23.7034, -57.9743)
  line L680 (-23.7034, -57.9743) -> (-18.1942, -59.3909)
  line L681 (-18.1942, -59.3909) -> (-12.4848, -60.2618)
  line L682 (-12.4848, -60.2618) -> (-8.0751, -60.5595)
  line L683 (-8.0751, -60.5595) -> (-6.6047, -60.5595)
  line L684 (-6.6047, -60.5595) -> (-6.6034, -60.5595)
  line L685 (-6.6034, -60.5595) -> (-5.1343, -60.5595)
  line L686 (-5.1343, -60.5595) -> (-0.7246, -60.2618)
  line L687 (-0.7246, -60.2618) -> (4.9843, -59.3909)
  line L688 (4.9843, -59.3909) -> (10.4941, -57.9743)
  line L689 (10.4941, -57.9743) -> (15.7773, -56.0395)
  line L690 (15.7773, -56.0395) -> (20.8029, -53.6183)
  line L691 (20.8029, -53.6183) -> (25.5449, -50.7382)
  line L692 (25.5449, -50.7382) -> (29.9713, -47.4282)
  line L693 (29.9713, -47.4282) -> (34.0544, -43.7171)
  line L694 (34.0544, -43.7171) -> (37.7653, -39.634)
  line L695 (37.7653, -39.634) -> (41.0754, -35.2076)
  line L696 (41.0754, -35.2076) -> (43.9553, -30.466)
  line L697 (43.9553, -30.466) -> (46.3769, -25.4401)
  line L698 (46.3769, -25.4401) -> (48.3114, -20.1569)
  line L699 (48.3114, -20.1569) -> (49.7282, -14.6473)
  line L700 (49.7282, -14.6473) -> (50.5989, -8.9382)
  line L701 (50.5989, -8.9382) -> (50.8966, -4.5285)
  line L702 (50.8966, -4.5285) -> (50.8966, -3.0596)
  line L703 (50.8966, -3.0596) -> (50.8966, -1.5892)
  line L704 (50.8966, -1.5892) -> (50.5989, 2.8205)
  line L705 (50.5989, 2.8205) -> (49.7282, 8.5299)
  line L706 (49.7282, 8.5299) -> (48.3114, 14.0407)
  line L707 (48.3114, 14.0407) -> (46.3769, 19.3229)
  line L708 (46.3769, 19.3229) -> (43.9553, 24.3498)
  line L709 (43.9553, 24.3498) -> (41.0754, 29.0902)
  line L710 (41.0754, 29.0902) -> (37.7653, 33.5164)
  line L711 (37.7653, 33.5164) -> (34.0544, 37.5994)
  line L712 (34.0544, 37.5994) -> (29.9713, 41.3106)
  line L713 (29.9713, 41.3106) -> (25.5449, 44.6205)
  line L714 (25.5449, 44.6205) -> (20.8029, 47.5009)
  line L715 (20.8029, 47.5009) -> (15.7773, 49.9235)
  line L716 (15.7773, 49.9235) -> (10.4941, 51.8567)
  line L717 (10.4941, 51.8567) -> (4.9843, 53.2735)
  line L718 (4.9843, 53.2735) -> (-0.7246, 54.1445)
  line L719 (-0.7246, 54.1445) -> (-5.1343, 54.4404)
  line L720 (-5.1343, 54.4404) -> (-6.6034, 54.4404)
  line L721 (-25.5447, 55.5374) -> (-25.7291, 55.2507)
  line L722 (-25.7291, 55.2507) -> (-26.4858, 54.5176)
  line L723 (-26.4858, 54.5176) -> (-27.6831, 53.8961)
  line L724 (-27.6831, 53.8961) -> (-29.0184, 53.7117)
  line L725 (-29.0184, 53.7117) -> (-30.0588, 53.8727)
  line L726 (-30.0588, 53.8727) -> (-30.3732, 54.001)
  line L727 (-30.3732, 54.001) -> (-30.9051, 54.2189)
  line L728 (-30.9051, 54.2189) -> (-32.5424, 54.7726)
  line L729 (-32.5424, 54.7726) -> (-35.2251, 55.4356)
  line L730 (-35.2251, 55.4356) -> (-38.3727, 55.8448)
  line L731 (-38.3727, 55.8448) -> (-41.0473, 55.9083)
  line L732 (-41.0473, 55.9083) -> (-41.932, 55.8491)
  line L733 (-41.932, 55.8491) -> (-42.708, 55.798)
  line L734 (-42.708, 55.798) -> (-45.0229, 55.4536)
  line L735 (-45.0229, 55.4536) -> (-48.0204, 54.6954)
  line L736 (-48.0204, 54.6954) -> (-50.8921, 53.604)
  line L737 (-50.8921, 53.604) -> (-53.6055, 52.2042)
  line L738 (-53.6055, 52.2042) -> (-56.1273, 50.5258)
  line L739 (-56.1273, 50.5258) -> (-58.4231, 48.5948)
  line L740 (-58.4231, 48.5948) -> (-60.4612, 46.4397)
  line L741 (-60.4612, 46.4397) -> (-61.809, 44.6992)
  line L742 (-61.809, 44.6992) -> (-62.2072, 44.0861)
  line L743 (-62.2072, 44.0861) -> (-62.994, 42.8788)
  line L744 (-62.994, 42.8788) -> (-64.9784, 39.0119)
  line L745 (-64.9784, 39.0119) -> (-66.5742, 34.0386)
  line L746 (-66.5742, 34.0386) -> (-67.0648, 28.9497)
  line L747 (-67.0648, 28.9497) -> (-66.7685, 24.8664)
  line L748 (-66.7685, 24.8664) -> (-66.5246, 23.5311)
  line L749 (-66.5246, 23.5311) -> (-66.3937, 22.805)
  line L750 (-66.3937, 22.805) -> (-65.8728, 20.6482)
  line L751 (-65.8728, 20.6482) -> (-65.1465, 18.3688)
  line L752 (-65.1465, 18.3688) -> (-64.4548, 16.6894)
  line L753 (-64.4548, 16.6894) -> (-64.0524, 15.8639)
  line L754 (-64.0524, 15.8639) -> (-63.9036, 15.5964)
  line L755 (-63.9036, 15.5964) -> (-63.8581, 15.5152)
  line L756 (-63.8581, 15.5152) -> (-63.8223, 15.0752)
  line L757 (-63.8223, 15.0752) -> (-64.0248, 14.6828)
  line L758 (-64.0248, 14.6828) -> (-64.0979, 14.6234)
  line L759 (-64.0979, 14.6234) -> (-64.1902, 14.5505)
  line L760 (-64.1902, 14.5505) -> (-64.7166, 14.4679)
  line L761 (-64.7166, 14.4679) -> (-65.1796, 14.7311)
  line L762 (-65.1796, 14.7311) -> (-65.2389, 14.8316)
  line L763 (-65.2389, 14.8316) -> (-65.4677, 15.2203)
  line L764 (-65.4677, 15.2203) -> (-66.1029, 16.4123)
  line L765 (-66.1029, 16.4123) -> (-67.1764, 18.7369)
  line L766 (-67.1764, 18.7369) -> (-68.2499, 21.6942)
  line L767 (-68.2499, 21.6942) -> (-68.9513, 24.2916)
  line L768 (-68.9513, 24.2916) -> (-69.1153, 25.1697)
  line L769 (-69.1153, 25.1697) -> (-69.2242, 25.7498)
  line L770 (-69.2242, 25.7498) -> (-69.4708, 27.5027)
  line L771 (-69.4708, 27.5027) -> (-69.6734, 30.077)
  line L772 (-69.6734, 30.077) -> (-69.6706, 32.8606)
  line L773 (-69.6706, 32.8606) -> (-69.4088, 35.8219)
  line L774 (-69.4088, 35.8219) -> (-68.8369, 38.9309)
  line L775 (-68.8369, 38.9309) -> (-67.8999, 42.1567)
  line L776 (-67.8999, 42.1567) -> (-66.5439, 45.4668)
  line L777 (-66.5439, 45.4668) -> (-65.2182, 48.016)
  line L778 (-65.2182, 48.016) -> (-64.7166, 48.829)
  line L779 (-64.7166, 48.829) -> (-64.0689, 49.8821)
  line L780 (-64.0689, 49.8821) -> (-61.802, 52.842)
  line L781 (-61.802, 52.842) -> (-58.5375, 56.1219)
  line L782 (-58.5375, 56.1219) -> (-55.0359, 58.7277)
  line L783 (-55.0359, 58.7277) -> (-51.4061, 60.7134)
  line L784 (-51.4061, 60.7134) -> (-47.757, 62.1369)
  line L785 (-27.4309, 61.3693) -> (-27.0288, 61.2138)
  line L786 (-27.0288, 61.2138) -> (-25.9648, 60.3716)
  line L787 (-25.9648, 60.3716) -> (-25.1091, 58.9027)
  line L788 (-25.1091, 58.9027) -> (-24.9435, 57.209)
  line L789 (-24.9435, 57.209) -> (-25.3115, 55.9027)
  line L790 (-25.3115, 55.9027) -> (-25.5447, 55.5374)
  line L791 (28.0803, 62.5295) -> (29.3579, 60.924)
  line L792 (29.3579, 60.924) -> (30.3351, 59.6784)
  line L793 (30.3351, 59.6784) -> (30.7854, 59.0858)
  line L794 (30.7854, 59.0858) -> (30.8837, 58.9441)
  line L795 (30.8837, 58.9441) -> (31.0457, 58.7056)
  line L796 (31.0457, 58.7056) -> (31.1727, 58.5181)
  line L797 (31.1727, 58.5181) -> (31.556, 57.952)
  line L798 (31.556, 57.952) -> (32.1733, 57.0078)
  line L799 (32.1733, 57.0078) -> (32.8278, 55.9454)
  line L800 (32.8278, 55.9454) -> (33.4478, 54.8361)
  line L801 (33.4478, 54.8361) -> (33.9619, 53.7543)
  line L802 (33.9619, 53.7543) -> (34.2982, 52.7704)
  line L803 (34.2982, 52.7704) -> (34.3876, 51.9573)
  line L804 (34.3876, 51.9573) -> (34.2568, 51.4887)
  line L805 (34.2568, 51.4887) -> (34.1578, 51.3868)
  line L806 (34.1578, 51.3868) -> (34.1468, 51.3744)
  line L807 (34.1468, 51.3744) -> (34.0435, 51.2738)
  line L808 (34.0435, 51.2738) -> (33.5692, 51.1387)
  line L809 (33.5692, 51.1387) -> (32.7519, 51.2227)
  line L810 (32.7519, 51.2227) -> (31.7656, 51.5565)
  line L811 (31.7656, 51.5565) -> (30.6807, 52.0691)
  line L812 (30.6807, 52.0691) -> (29.5715, 52.6878)
  line L813 (29.5715, 52.6878) -> (28.5075, 53.3408)
  line L814 (28.5075, 53.3408) -> (27.5637, 53.9581)
  line L815 (27.5637, 53.9581) -> (26.9988, 54.3413)
  line L816 (26.9988, 54.3413) -> (26.8116, 54.4683)
  line L817 (26.8116, 54.4683) -> (26.5715, 54.6319)
  line L818 (26.5715, 54.6319) -> (26.4298, 54.7287)
  line L819 (26.4298, 54.7287) -> (25.84, 55.1778)
  line L820 (25.84, 55.1778) -> (24.5982, 56.1521)
  line L821 (24.5982, 56.1521) -> (22.9983, 57.4252)
  line L822 (22.9983, 57.4252) -> (21.645, 58.5072)
  line L823 (21.645, 58.5072) -> (21.1946, 58.8666)
  line L824 (21.1946, 58.8666) -> (20.7565, 59.2181)
  line L825 (20.7565, 59.2181) -> (18.123, 61.2936)
  line L826 (51.9108, -39.6367) -> (51.9136, -39.6395)
  line L827 (51.9136, -39.6395) -> (51.9494, -39.6753)
  line L828 (51.9494, -39.6753) -> (51.9535, -39.6794)
  line L829 (51.9535, -39.6794) -> (52.3106, -40.0336)
  line L830 (52.3106, -40.0336) -> (53.0797, -41.4047)
  line L831 (53.0797, -41.4047) -> (53.3883, -43.3533)
  line L832 (53.3883, -43.3533) -> (52.8852, -45.2508)
  line L833 (52.8852, -45.2508) -> (51.9715, -46.5228)
  line L834 (51.9715, -46.5228) -> (51.5761, -46.8301)
  line L835 (51.5761, -46.8301) -> (51.0152, -47.2642)
  line L836 (51.0152, -47.2642) -> (48.1417, -49.5035)
  line L837 (48.1417, -49.5035) -> (45.5154, -51.5747)
  line L838 (45.5154, -51.5747) -> (45.0787, -51.9247)
  line L839 (45.0787, -51.9247) -> (44.6253, -52.2857)
  line L840 (44.6253, -52.2857) -> (43.2664, -53.3716)
  line L841 (43.2664, -53.3716) -> (41.6609, -54.6491)
  line L842 (41.6609, -54.6491) -> (40.4153, -55.6261)
  line L843 (40.4153, -55.6261) -> (39.824, -56.0767)
  line L844 (39.824, -56.0767) -> (39.6823, -56.1746)
  line L845 (39.6823, -56.1746) -> (39.4437, -56.3372)
  line L846 (39.4437, -56.3372) -> (39.255, -56.4639)
  line L847 (39.255, -56.4639) -> (38.6889, -56.8457)
  line L848 (38.6889, -56.8457) -> (37.7447, -57.4644)
  line L849 (37.7447, -57.4644) -> (36.6823, -58.119)
  line L850 (36.6823, -58.119) -> (35.5741, -58.7377)
  line L851 (35.5741, -58.7377) -> (34.491, -59.2517)
  line L852 (34.491, -59.2517) -> (33.5073, -59.5894)
  line L853 (33.5073, -59.5894) -> (32.694, -59.6789)
  line L854 (32.694, -59.6789) -> (32.2256, -59.5466)
  line L855 (32.2256, -59.5466) -> (32.125, -59.4488)
  line L856 (32.125, -59.4488) -> (32.1125, -59.4378)
  line L857 (32.1125, -59.4378) -> (31.9198, -59.2393)
  line L858 (31.9198, -59.2393) -> (31.9609, -58.0432)
  line L859 (31.9609, -58.0432) -> (32.8072, -55.972)
  line L860 (32.8072, -55.972) -> (34.079, -53.7988)
  line L861 (34.079, -53.7988) -> (34.9198, -52.5228)
  line L862 (34.9198, -52.5228) -> (35.2063, -52.1025)
  line L863 (35.2063, -52.1025) -> (35.3701, -51.8627)
  line L864 (35.3701, -51.8627) -> (35.4669, -51.7208)
  line L865 (35.4669, -51.7208) -> (35.9159, -51.1309)
  line L866 (35.9159, -51.1309) -> (36.8903, -49.8893)
  line L867 (36.8903, -49.8893) -> (38.1621, -48.2894)
  line L868 (38.1621, -48.2894) -> (39.2454, -46.9362)
  line L869 (39.2454, -46.9362) -> (39.6063, -46.4856)
  line L870 (39.6063, -46.4856) -> (39.9563, -46.0474)
  line L871 (39.9563, -46.0474) -> (42.0318, -43.4139)
  line L872 (42.0318, -43.4139) -> (44.2779, -40.5311)
  line L873 (44.2779, -40.5311) -> (44.715, -39.9688)
  line L874 (44.715, -39.9688) -> (45.0208, -39.5734)
  line L875 (45.0208, -39.5734) -> (46.2911, -38.6582)
  line L876 (46.2911, -38.6582) -> (48.1902, -38.1553)
  line L877 (48.1902, -38.1553) -> (50.1389, -38.4642)
  line L878 (50.1389, -38.4642) -> (51.5098, -39.2329)
  line L879 (51.5098, -39.2329) -> (51.8654, -39.5913)
  line L880 (51.8654, -39.5913) -> (51.8682, -39.594)
  line L881 (51.8682, -39.594) -> (51.9068, -39.6326)
  line L882 (51.9068, -39.6326) -> (51.9108, -39.6367)
  line L883 (-13.5984, -9.5235) -> (0.2855, 4.3586)
  line L884 (-12.8913, -10.2307) -> (0.9926, 3.6514)
  line L885 (-0.3189, -10.2315) -> (-14.2011, 3.6524)
  line L886 (0.3882, -9.5245) -> (-13.4939, 4.3594)
  line L887 (0.9926, 3.6514) -> (0.2855, 4.3586)
  line L888 (0.3882, -9.5245) -> (-0.3189, -10.2315)
  line L889 (-13.4939, 4.3594) -> (-14.2011, 3.6524)
  line L890 (-12.8913, -10.2307) -> (-13.5984, -9.5235)
  point P0 (0, 0)
  point P1 (-6.6047, -2.5307)
  point P2 (-7.3118, -3.2377)
  point P3 (-6.6048, -3.9449)
  point P4 (-5.8976, -3.2378)
  dimension "d4" = 0.5
  dimension "d5" = 0.5
  dimension "d6" = 0.5
  dimension "d7" = 0.5
  constraints: 1782 end point, 5 parallel, 3 perpendicular
  measures "d4" distance between parallel lines of L240 L883
  measures "d5" distance between parallel lines of L240 L884
  measures "d6" distance between parallel lines of L243 L885
  measures "d7" distance between parallel lines of L243 L886